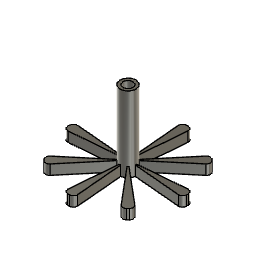
Chair v14 (Autodesk Fusion 360 archive; units mm, degrees)
design "wheel base"
Autodesk Fusion 360 part; units mm, degrees
sketch "Sketch1" plane through (0, 0, 0) normal (0, 0, 1) x (1, 0, 0)
  circle A0 centre (0, 0) radius 40
  line L0 (39.8478, 3.4862) -> (278.222, 24.3413)
  line L1 (0, 0) -> (300, 0) construction
  line L2 (39.8478, -3.4862) -> (278.222, -24.3413)
  arc A1 (299.9627, -4.7329) -> (299.9627, 4.7329) centre (0, 0) ccw
  arc A2 (299.9627, 4.7329) -> (278.222, 24.3413) centre (279.9652, 4.4174) ccw
  arc A3 (278.222, -24.3413) -> (299.9627, -4.7329) centre (279.9652, -4.4174) ccw
  line L3 (25.7115, 30.6418) -> (179.5208, 213.9446)
  line L4 (30.6418, 25.7115) -> (213.9446, 179.5208)
  arc A4 (213.9446, 179.5208) -> (215.4523, 208.759) centre (201.0888, 194.8417) ccw
  arc A5 (215.4523, 208.759) -> (208.759, 215.4523) centre (0, 0) ccw
  arc A6 (208.759, 215.4523) -> (179.5208, 213.9446) centre (194.8417, 201.0888) ccw
  line L5 (-3.4862, 39.8478) -> (-24.3413, 278.222)
  line L6 (3.4862, 39.8478) -> (24.3413, 278.222)
  arc A7 (24.3413, 278.222) -> (4.7329, 299.9627) centre (4.4174, 279.9652) ccw
  arc A8 (4.7329, 299.9627) -> (-4.7329, 299.9627) centre (0, 0) ccw
  arc A9 (-4.7329, 299.9627) -> (-24.3413, 278.222) centre (-4.4174, 279.9652) ccw
  line L7 (-30.6418, 25.7115) -> (-213.9446, 179.5208)
  line L8 (-25.7115, 30.6418) -> (-179.5208, 213.9446)
  arc A10 (-179.5208, 213.9446) -> (-208.759, 215.4523) centre (-194.8417, 201.0888) ccw
  arc A11 (-208.759, 215.4523) -> (-215.4523, 208.759) centre (0, 0) ccw
  arc A12 (-215.4523, 208.759) -> (-213.9446, 179.5208) centre (-201.0888, 194.8417) ccw
  line L9 (-39.8478, -3.4862) -> (-278.222, -24.3413)
  line L10 (-39.8478, 3.4862) -> (-278.222, 24.3413)
  arc A13 (-278.222, 24.3413) -> (-299.9627, 4.7329) centre (-279.9652, 4.4174) ccw
  arc A14 (-299.9627, 4.7329) -> (-299.9627, -4.7329) centre (0, 0) ccw
  arc A15 (-299.9627, -4.7329) -> (-278.222, -24.3413) centre (-279.9652, -4.4174) ccw
  line L11 (-25.7115, -30.6418) -> (-179.5208, -213.9446)
  line L12 (-30.6418, -25.7115) -> (-213.9446, -179.5208)
  arc A16 (-213.9446, -179.5208) -> (-215.4523, -208.759) centre (-201.0888, -194.8417) ccw
  arc A17 (-215.4523, -208.759) -> (-208.759, -215.4523) centre (0, 0) ccw
  arc A18 (-208.759, -215.4523) -> (-179.5208, -213.9446) centre (-194.8417, -201.0888) ccw
  line L13 (3.4862, -39.8478) -> (24.3413, -278.222)
  line L14 (-3.4862, -39.8478) -> (-24.3413, -278.222)
  arc A19 (-24.3413, -278.222) -> (-4.7329, -299.9627) centre (-4.4174, -279.9652) ccw
  arc A20 (-4.7329, -299.9627) -> (4.7329, -299.9627) centre (0, 0) ccw
  arc A21 (4.7329, -299.9627) -> (24.3413, -278.222) centre (4.4174, -279.9652) ccw
  line L15 (30.6418, -25.7115) -> (213.9446, -179.5208)
  line L16 (25.7115, -30.6418) -> (179.5208, -213.9446)
  arc A22 (179.5208, -213.9446) -> (208.759, -215.4523) centre (194.8417, -201.0888) ccw
  arc A23 (208.759, -215.4523) -> (215.4523, -208.759) centre (0, 0) ccw
  arc A24 (215.4523, -208.759) -> (213.9446, -179.5208) centre (201.0888, -194.8417) ccw
  point P0 (298.8584, 26.1467)
  dimension "d1" = 80
  dimension "d3" = 5
  dimension "d4" = 300
  dimension "d5" = 20
  dimension "d6" = 20
  dimension "d8" = 360
  constraint coincident A0.centre L1.start
  constraint concentric A0 A1
  constraint horizontal L1
  constraint coincident A0 L0.start
  constraint coincident A0 L2.start
  constraint coincident P0 L0
  constraint tangent L0 A2
  constraint tangent A1 A2
  constraint tangent L2 A3
  constraint tangent A1 A3
  measures "d1" diameter of A0
  measures "d3" angle of L0 L1
  measures "d4" distance of A0.centre P0
  measures "d5" radius of A2
  measures "d6" radius of A3
extrude "Extrude1" add sketch "Sketch1" along normal blind 50 contours A0 L0 L2 A1 A2 A3 | A0 L3 L4 A4 A5 A6 | A0 L15 L16 A22 A23 A24 | A0 L5 L6 A7 A8 A9 | A0 L13 L14 A19 A20 A21 | A0 L7 L8 A10 A11 A12 | A0 L11 L12 A16 A17 A18 | A0 L9 L10 A13 A14 A15 makes body 1 at (-10.4379, 119.3059, 16.6667) makes body 2 at (10.4379, -119.3059, 16.6667) makes body 3 at (-76.9813, -91.7427, 16.6667) makes body 4 at (91.7427, 76.9813, 16.6667) makes body 5 at (-91.7427, 76.9813, 16.6667) makes body 6 at (76.9813, -91.7427, 16.6667) makes body 7 at (-119.3059, -10.4379, 16.6667) makes body 8 at (119.3059, 10.4379, 16.6667)
extrude "Extrude2" add sketch "Sketch1" along normal blind 80 contours A0 bodies 1 2 3 4 5 6 7 8
extrude "Extrude3" add 1 faces at (13.1844, -1.9872, 80) along direction (0, 0, 1) blind 300 on bodies 1 bodies 1
sketch "Sketch2" plane through (0, 0, 380) normal (0, 0, 1) x (-1, 0, 0)
  circle A0 centre (0, 0) radius 40
  circle A1 centre (0, 0) radius 25
  dimension "d15" = 50
  constraint coincident A0.centre A1.centre
  measures "d15" diameter of A1
extrude "Extrude4" cut sketch "Sketch2" against normal blind 280 contours A1 bodies 1

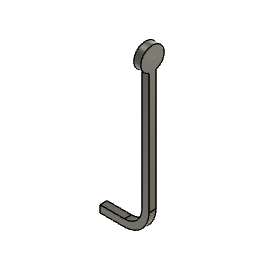
design "back link"
Autodesk Fusion 360 part; units mm, degrees
sketch "Sketch1" plane through (0, 0, 0) normal (1, 0, 0) x (0, 1, 0)
  line L0 (7.5, -7.5) -> (-7.5, -7.5)
  line L1 (-7.5, -7.5) -> (-7.5, 7.5)
  line L2 (-7.5, 7.5) -> (7.5, 7.5)
  line L3 (7.5, 7.5) -> (7.5, -7.5)
  line L4 (7.5, -7.5) -> (-7.5, 7.5) construction
  line L5 (-7.5, -7.5) -> (7.5, 7.5) construction
  dimension "d1" = 15
  dimension "d2" = 15
  constraint horizontal L0
  constraint perpendicular L0 L1
  constraint parallel L0 L2
  constraint parallel L1 L3
  constraint coincident L4 origin
  constraint coincident L5 origin
  measures "d1" distance of L1.end L2.end
  measures "d2" distance of L0.end L1.end
sketch "Sketch2" plane through (0, 0, 0) normal (0, 1, 0) x (1, 0, 0)
  line L0 (0, -7.5) -> (52.5, -7.5)
  line L1 (90, -45) -> (90, -257.5)
  arc A0 (90, -45) -> (52.5, -7.5) centre (52.5, -45) ccw
  point P0 (90, -7.5)
  dimension "d3" = 7.5
  dimension "d4" = 90
  dimension "d5" = 250
  dimension "d6" = 37.5
  constraint perpendicular L0 L1
  constraint coincident P0 L1
  constraint coincident P0 L0
  constraint tangent L1 A0
  constraint tangent L0 A0
  measures "d3" distance of origin L0.start
  measures "d4" distance of L0.start P0
  measures "d5" distance of P0 L1.end
  measures "d6" radius of A0
sweep "Sweep1" add profiles "Sketch1" path "Sketch2" along L1 A0 L0 section 1
extrude "Extrude1" add 1 faces at (95, 2.5, 257.5) along direction (0, 0, 1) blind 50
extrude "Extrude2" add 1 faces at (95, 2.5, 307.5) along direction (0, 0, 1) blind 20
ref_plane "WorkPlane1" through (90, 7.5, 327.5) normal (1, 0, 0) x (0, 1, 0)
sketch "Sketch4" plane through (0, 0, 327.5) normal (0, 0, 1) x (-1, 0, 0)
  line L0 (-90, -7.5) -> (-90, 7.5)
  line L1 (-90, 7.5) -> (-105, 7.5)
  line L2 (-105, 7.5) -> (-105, -7.5)
  line L3 (-105, -7.5) -> (-90, -7.5)
sketch "Sketch3" plane through (90, 7.5, 327.5) normal (1, 0, 0) x (0, 1, 0)
  circle A0 centre (-7.5, 0) radius 25
  point P0 (-7.5, 0)
  dimension "d17" = 50
  constraint coincident P0 A0.centre
  measures "d17" diameter of A0
extrude "Extrude3" add sketch "Sketch3" along normal blind 15

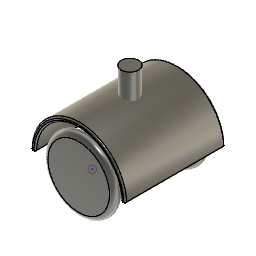
design "Wheel"
Autodesk Fusion 360 part; units mm, degrees
sketch "Sketch1" plane through (0, 0, 0) normal (0, 0, 1) x (1, 0, 0)
sketch "Sketch2" plane through (0, 0, 0) normal (0, 1, 0) x (1, 0, 0)
  circle A0 centre (0, 0) radius 10
  dimension "d1" = 20
  constraint coincident A0.centre origin
  measures "d1" diameter of A0
extrude "Extrude1" add sketch "Sketch2" along normal blind 50 makes body 1
sketch "Sketch3" plane through (0, 0, 0) normal (0, -1, 0) x (1, 0, 0)
  circle A0 centre (0, 0) radius 10
  circle A1 centre (0, 0) radius 7.5
  dimension "d4" = 15
  constraint coincident A0.centre A1.centre
  measures "d4" diameter of A1
extrude "Extrude2" cut sketch "Sketch3" against normal blind 145 contours A1 bodies 1
sketch "Sketch4" plane through (0, 0, 0) normal (0, 1, 0) x (1, 0, 0)
sketch "Sketch1 (2)" plane through (0, 0, 0) normal (0, 1, 0) x (1, 0, 0) in component "Component"
  circle A0 centre (0, 0) radius 25
  constraint coincident A0.centre origin
extrude "Extrude1'" add sketch "Sketch1 (2)" against normal blind 7 separate body makes body 2 in component "Component"
fillet "Fillet1" radius 3.5 2 edges at (-23.3082, -7, -9.0404) (-23.3082, 0, 9.0404) on bodies 2 in component "Component"
copy_body "CopyPasteBodies1" bodies 2 makes body 3
move_body "Move1" bodies 3 to x (1, 0, 0) y (0, 1, 0) z (0, 0, 1) at (0, 130, 0)
move_body "Align1" bodies 3 to x (1, 0, 0) y (0, 1, 0) z (0, 0, 1) at (0, -73, 0)
sketch "Sketch1 (3)" plane through (0, 0, 0) normal (0, 1, 0) x (1, 0, 0) in component "Component'"
  circle A0 centre (0, 0) radius 6
  dimension "d12" = 12
  constraint coincident A0.centre origin
  measures "d12" diameter of A0
extrude "Extrude1''" add sketch "Sketch1 (3)" along normal blind 55 separate body makes body 4 in component "Component'"
move_body "Move2" bodies 3 to x (1, 0, 0) y (0, 1, 0) z (0, 0, 1) at (0, 50, 0)
copy_body "Body->Comp1" bodies 3 removing the originals makes body 5 in component "Component''"
ref_plane "WorkPlane1" through (0, 0, 50) normal (0, 0, 1) x (1, 0, 0)
sketch "Sketch6" plane through (0, 0, 50) normal (0, 0, 1) x (1, 0, 0)
  circle A0 centre (0.1118, 26.2789) radius 6
  dimension "d25" = 12
  measures "d25" diameter of A0
extrude "Extrude3" add sketch "Sketch6" along normal up to surface end surface at (9.9503, 16.6667, 0.9957) on bodies 1 bodies 1
ref_plane "WorkPlane2" through (0, 60, 0) normal (0, 1, 0) x (0, 0, 1)
sketch "Sketch7" plane through (0, 60, 0) normal (0, 1, 0) x (1, 0, 0)
  arc A0 (-30, 0) -> (30, 0) centre (0, 0) ccw
  constraint coincident A0.centre origin
surface "Extrude4" add extruded along (0, 1, 0) between 0 and -70 path "Sketch7" along A0 separate body makes body 6
thicken "Thicken1" add thickness 3 1 faces at (23.914, 36.6667, 18.1141) separate body on bodies 6 makes body 7
fillet "Fillet1'" radius 1 2 edges at (0, 60, 33) (0, 60, 30) on bodies 7
fillet "Fillet2" radius 1 2 edges at (0, -10, 33) (0, -10, 30) on bodies 7
fillet "Fillet3" radius 1 8 edges at (32.7071, -9.7071, 0) (31.5, -10, 0) (30.2929, -9.7071, 0) (30, 25, 0) (30.2929, 59.7071, 0) (31.5, 60, 0) (32.7071, 59.7071, 0) (33, 25, 0) on bodies 7
fillet "Fillet4" radius 1 8 edges at (-31.5, -10, 0) (-30.2929, -9.7071, 0) (-30, 25, 0) (-30.2929, 59.7071, 0) (-31.5, 60, 0) (-32.7071, 59.7071, 0) (-33, 25, 0) (-32.7071, -9.7071, 0) on bodies 7
extrude "Extrude5" add 1 faces at (9.1015, 50, 0.8694) along direction (0, 1, 0) up to surface (2.5 mm away) on bodies 1 bodies 1
component "Component" placed x (1, 0, 0) y (0, 1, 0) z (0, 0, 1) at (0, -2.5, 0)
component "Component'" placed x (1, 0, 0) y (0, 1, 0) z (0, 0, 1) at (0, -2.5, 0)
component "Component''" placed x (1, 0, 0) y (0, 1, 0) z (0, 0, 1) at (0, -47.5, 0)
hidden bodies 6
